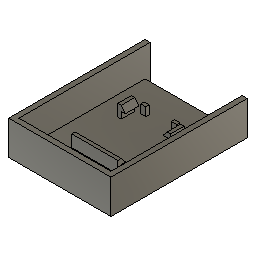
Uni-stick holder joystick-A (Autodesk Fusion 360 design; units mm, degrees)
Autodesk Fusion 360 part; units mm, degrees
note: some values were not read from the file. Set by a fixed rule: which sketch regions a step uses.
sketch "Sketch1" plane through (0, 0, 0) normal (0, 0, 1) x (1, 0, 0)
  line L0 (30, -40) -> (-30, -40)
  line L1 (-30, -40) -> (-30, 40)
  line L2 (-27, 40) -> (27, 40)
  line L3 (30, 40) -> (30, -40)
  line L4 (30, -40) -> (-30, 40) construction
  line L5 (-30, -40) -> (30, 40) construction
  line L6 (27, -37) -> (-27, -37)
  line L7 (-27, -37) -> (-27, 37)
  line L8 (-27, 37) -> (27, 37)
  line L9 (27, 37) -> (27, -37)
  line L10 (27, 37) -> (27, 40)
  line L11 (-27, 37) -> (-27, 40)
  line L12 (27, 40) -> (30, 40)
  line L13 (-30, 40) -> (-27, 40)
  line L14 (13.5, 17.5) -> (-13.5, 17.5)
  line L15 (-13.5, 17.5) -> (-13.5, -17.5)
  line L16 (-13.5, -17.5) -> (13.5, -17.5)
  line L17 (13.5, -17.5) -> (13.5, 17.5)
  line L18 (13.5, 17.5) -> (-13.5, -17.5) construction
  line L19 (-13.5, 17.5) -> (13.5, -17.5) construction
  line L20 (-13.5, -17.5) -> (13.5, -17.5)
  line L21 (13.5, -17.5) -> (13.5, -19.5)
  line L22 (13.5, -19.5) -> (-13.5, -19.5)
  line L23 (-13.5, -19.5) -> (-13.5, -17.5)
  line L24 (13.5, 17.5) -> (15.5, 17.5)
  line L25 (15.5, 17.5) -> (15.5, 9.5)
  line L26 (15.5, 9.5) -> (13.5, 9.5)
  line L27 (13.5, 9.5) -> (13.5, 17.5)
  line L28 (-13.5, 17.5) -> (-15.5, 17.5)
  line L29 (-15.5, 17.5) -> (-15.5, 9.5)
  line L30 (-15.5, 9.5) -> (-13.5, 9.5)
  line L31 (-13.5, 9.5) -> (-13.5, 17.5)
  line L32 (7.5, 18) -> (10.5, 18)
  line L33 (10.5, 18) -> (10.5, 20)
  line L34 (10.5, 20) -> (7.5, 20)
  line L35 (7.5, 20) -> (7.5, 18)
  line L36 (7.5, 18) -> (10.5, 20) construction
  line L37 (10.5, 18) -> (7.5, 20) construction
  line L38 (0, 10) -> (0, 29)
  line L39 (-7.5, 20) -> (-7.5, 18)
  line L40 (-10.5, 20) -> (-7.5, 20)
  line L41 (-7.5, 18) -> (-10.5, 18)
  line L42 (-7.5, 18) -> (-10.5, 20) construction
  line L43 (-10.5, 18) -> (-10.5, 20)
  line L44 (-10.5, 18) -> (-7.5, 20) construction
  point P0 (9, 19)
  point P1 (-9, 19)
  dimension "d1" = 60
  dimension "d2" = 80
  dimension "d8" = 27
  dimension "d9" = 35
  dimension "d10" = 2
  dimension "d11" = 2
  dimension "d12" = 8
  dimension "d13" = 2
  dimension "d14" = 8
  dimension "d24" = 3
  dimension "d25" = 2
  constraint horizontal L0
  constraint perpendicular L0 L1
  constraint parallel L0 L2
  constraint parallel L1 L3
  constraint coincident L4 origin
  constraint coincident L5 origin
  constraint perpendicular L2 L10
  constraint perpendicular L2 L11
  constraint parallel L0 L12
  constraint coincident L2.start L12
  constraint horizontal L14
  constraint perpendicular L14 L15
  constraint parallel L14 L16
  constraint parallel L15 L17
  constraint coincident L18 origin
  constraint coincident L19 origin
  constraint horizontal L20
  constraint vertical L21
  constraint horizontal L22
  constraint vertical L23
  constraint collinear L17 L21
  constraint horizontal L24
  constraint vertical L25
  constraint horizontal L26
  constraint vertical L27
  constraint horizontal L28
  constraint vertical L29
  constraint horizontal L30
  constraint vertical L31
  constraint horizontal L32
  constraint perpendicular L32 L33
  constraint parallel L32 L34
  constraint parallel L33 L35
  constraint coincident L36 P0
  constraint coincident L37 P0
  constraint vertical L38
  constraint symmetric L32.start L38 L39.end
  constraint symmetric L32.end L38 L41.end
  constraint symmetric L33.end L38 L40.start
  constraint symmetric L34.end L38 L39.start
  constraint symmetric P0 L38 P1
  measures "d1" distance of L1.end L3.start
  measures "d2" distance of L0.end L1.end
  measures "d8" distance of L15.end L16.end
  measures "d9" distance of L14.end L15.end
  measures "d10" distance of L15.end L22.end
  measures "d11" distance of L14.start L24.end
  measures "d12" distance of L14.start L26.end
  measures "d13" distance of L14.end L28.end
  measures "d14" distance of L14.end L30.end
  measures "d24" distance of L33.end L34.end
  measures "d25" distance of L32.end L33.end
extrude "Extrude1" add sketch "Sketch1" along normal blind 3 contours L6 L7 L8 L9 | L14 L15 L16 L17 L20 L27 L31 | L17 L24 L25 L26 L27 | L15 L28 L29 L30 L31 | L16 L20 L21 L22 L23 | L32 L33 L34 L35 | L39 L40 L41 L43
extrude "Extrude2" add sketch "Sketch1" along normal blind 20 contours L0 L1 L3 L6 L7 L9 L10 L11 L12 L13
extrude "Extrude3" add sketch "Sketch1" along normal blind 10 contours L17 L24 L25 L26 L27 | L15 L28 L29 L30 L31 | L16 L20 L21 L22 L23
ref_plane "WorkPlane1" through (14.5, 13.5, 7) normal (0, 0, 1) x (1, 0, 0)
sketch "Sketch2" plane through (0, 0, 7) normal (0, 0, 1) x (1, 0, 0)
  line L0 (15.5, 9.5) -> (13.5, 9.5)
  line L1 (15.5, 17.5) -> (15.5, 9.5)
  line L2 (13.5, 9.5) -> (13.5, 17.5)
  line L3 (13.5, 17.5) -> (15.5, 17.5)
  line L4 (-15.5, 17.5) -> (-15.5, 9.5)
  line L5 (-13.5, 9.5) -> (-13.5, 17.5)
  line L6 (-15.5, 9.5) -> (-13.5, 9.5)
  line L7 (-13.5, 17.5) -> (-15.5, 17.5)
  line L8 (-13.5, 9.5) -> (-13.5, 17.5)
  line L9 (-13.5, 17.5) -> (-15.5, 17.5)
  line L10 (-15.5, 17.5) -> (-15.5, 9.5)
  line L11 (-15.5, 9.5) -> (-13.5, 9.5)
  line L12 (-13.5, -17.5) -> (13.5, -17.5)
  line L13 (13.5, -19.5) -> (-13.5, -19.5)
  line L14 (13.5, -17.5) -> (13.5, -19.5)
  line L15 (-13.5, -19.5) -> (-13.5, -17.5)
  line L16 (15.5, 9.5) -> (11, 9.5)
  line L17 (11, 9.5) -> (11, 17.5)
  line L18 (11, 17.5) -> (15.5, 17.5)
  line L19 (15.5, 17.5) -> (15.5, 9.5)
  line L20 (-13.5, 9.5) -> (-11, 9.5)
  line L21 (-11, 9.5) -> (-11, 17.5)
  line L22 (-11, 17.5) -> (-13.5, 17.5)
  line L23 (-13.5, 17.5) -> (-13.5, 9.5)
  line L24 (13.5, -17.5) -> (-13.5, -17.5)
  line L25 (-13.5, -17.5) -> (-13.5, -15)
  line L26 (-13.5, -15) -> (13.5, -15)
  line L27 (13.5, -15) -> (13.5, -17.5)
  dimension "d18" = 4.5
  dimension "d19" = 8
  dimension "d20" = 2.5
  dimension "d21" = 8
  dimension "d22" = 27
  dimension "d23" = 2.5
  constraint horizontal L16
  constraint vertical L17
  constraint horizontal L18
  constraint vertical L19
  constraint coincident L0.start L1.end
  constraint horizontal L20
  constraint vertical L21
  constraint horizontal L22
  constraint vertical L23
  constraint coincident L5.start L6.end
  constraint horizontal L24
  constraint vertical L25
  constraint horizontal L26
  constraint vertical L27
  constraint coincident L12.end L14.start
  measures "d18" distance of L0.start L16.end
  measures "d19" distance of L0.start L1.start
  measures "d20" distance of L5.start L20.end
  measures "d21" distance of L5.start L5.end
  measures "d22" distance of L12.end L12.start
  measures "d23" distance of L12.end L26.end
loft "Loft1" add profiles "Sketch2" section 1 face at (-4.5, -18.1667, 10) section 2 contours L12 L24 L25 L26 L27 | L12 L13 L14 L15 L24
loft "Loft2" add profiles "Sketch2" section 1 face at (14.8333, 14.8333, 10) section 2 contours L0 L1 L2 L3 L16 L18 L19 | L2 L16 L17 L18
loft "Loft3" add profiles "Sketch2" section 1 face at (-14.1667, 12.1667, 10) section 2 contours L4 L5 L6 L7 L8 L9 L10 L11 L23 | L5 L8 L20 L21 L22 L23
extrude "Extrude4" add sketch "Sketch1" along normal blind 8 contours L32 L33 L34 L35 | L39 L40 L41 L43
